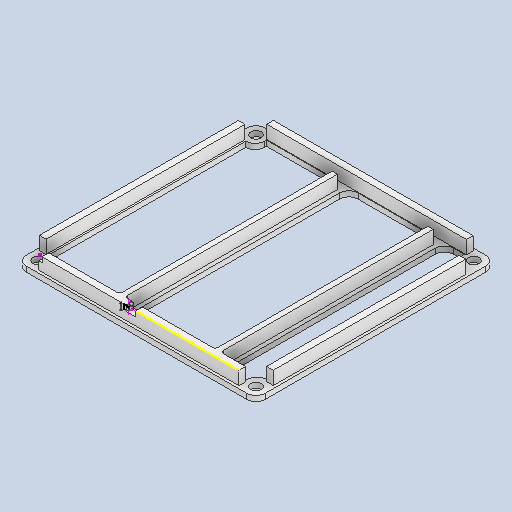
# Autodesk Inventor part: LeftCover
Saved by Autodesk Inventor 2024 (Build 280153000, 153)
## iProperties
Created: 2023-11-21
Part Number: LeftCover
Material: ABS Plastic
Document SubType Name: Modeling
Designer: G2O
Density: 1.06 g/cm^3
Appearance: Smooth - White
Author: G2O
Autodesk Inventor part; units mm, degrees
ref_plane "YZ Plane" through (0, 0, 0) normal (1, 0, 0) x (0, 1, 0)
ref_plane "XZ Plane" through (0, 0, 0) normal (0, 1, 0) x (-1, 0, 0)
ref_plane "XY Plane" through (0, 0, 0) normal (0, 0, 1) x (1, 0, 0)
sketch "Sketch1" plane through (0, 0, 0) normal (0, 1, 0) x (-1, 0, 0)
  line L0 (45, -45) -> (-45, -45)
  line L1 (-45, -45) -> (-45, 45)
  line L2 (-45, 45) -> (45, 45)
  line L3 (45, 45) -> (45, -45)
  line L4 (45, -45) -> (-45, 45) construction
  line L5 (-45, -45) -> (45, 45) construction
  point P0 (0, 0)
  dimension "d2" = 90
  dimension "d3" = 90
  constraints: 12 end point, 2 midpoint, 2 parallel, 1 horizontal, 1 perpendicular
  measures "d2" distance of L1.end L2.end
  measures "d3" distance of L0.end L1.end
extrude "Extrusion1" add sketch "Sketch1" along normal blind 2
sketch "Sketch2" plane through (0, 2, 0) normal (0, 1, 0) x (1, 0, 0)
  line L0 (45, -45) -> (45, 45) projected
  line L1 (45, 45) -> (41, 45)
  line L2 (45, 45) -> (-45, 45) projected
  circle A0 centre (41, 41) radius 2
  point P0 (0, 0)
  constraints: 2 end point, 1 centre point, 1 point on line
hole "Hole1" at (41, 2, -41) direction (0, -1, 0) diameter 4 end through all
sketch "Sketch3" plane through (0, 2, 0) normal (0, 1, 0) x (1, 0, 0)
  circle A0 centre (-41, 41) radius 2
  line L0 (-45, 45) -> (-45, -45) projected
  circle A1 centre (-41, -41) radius 2
  line L1 (45, -45) -> (45, 45) projected
  circle A2 centre (41, -41) radius 2
  point P0 (0, 0)
  dimension "d17" = 4
  dimension "d21" = 4
  constraints: 3 centre point
  measures "d17" diameter of A0
  measures "d21" diameter of A2
extrude "Extrusion2" cut sketch "Sketch3" against normal blind 2
fillet "Fillet1" radius 3.5 4 edges at (-45, 1, -45) (45, 1, -45) (45, 1, 45) (-45, 1, 45)
sketch "Sketch5" plane through (0, 2, 0) normal (0, 1, 0) x (1, 0, 0)
  line L0 (40, 40) -> (-40, 40)
  line L1 (-40, 40) -> (-40, -40)
  line L2 (-40, -40) -> (40, -40)
  line L3 (40, -40) -> (40, 40)
  line L4 (40, 40) -> (-40, -40) construction
  line L5 (-40, 40) -> (40, -40) construction
  line L6 (-9.8412, 41.25) -> (-37.3412, 41.25)
  line L7 (-37.3412, 41.25) -> (-37.3412, -41.25)
  line L8 (-37.3412, -41.25) -> (-9.8412, -41.25)
  line L9 (-9.8412, -41.25) -> (-9.8412, 41.25)
  line L10 (-9.8412, 41.25) -> (-37.3412, -41.25) construction
  line L11 (-37.3412, 41.25) -> (-9.8412, -41.25) construction
  line L12 (26.1588, 41.25) -> (-6.3412, 41.25)
  line L13 (-6.3412, 41.25) -> (-6.3412, -41.25)
  line L14 (-6.3412, -41.25) -> (26.1588, -41.25)
  line L15 (26.1588, -41.25) -> (26.1588, 41.25)
  line L16 (26.1588, 41.25) -> (-6.3412, -41.25) construction
  line L17 (-6.3412, 41.25) -> (26.1588, -41.25) construction
  line L18 (37.1268, 41.25) -> (29.6588, 41.25)
  line L19 (29.6588, 41.25) -> (29.6588, -41.25)
  line L20 (29.6588, -41.25) -> (37.1268, -41.25)
  line L21 (37.1268, -41.25) -> (37.1268, 41.25)
  line L22 (37.1268, 41.25) -> (29.6588, -41.25) construction
  line L23 (29.6588, 41.25) -> (37.1268, -41.25) construction
  line L24 (-41.5049, 41.25) -> (-37.5049, 41.25)
  line L25 (41.2164, 37.1336) -> (36.7164, 37.1336)
  line L26 (36.7164, 37.1336) -> (36.7164, -36.7164)
  line L27 (36.7164, -36.7164) -> (41.2164, -36.7164)
  line L28 (41.2164, -36.7164) -> (41.2164, 37.1336)
  line L29 (41.2164, 37.1336) -> (36.7164, -36.7164) construction
  line L30 (36.7164, 37.1336) -> (41.2164, -36.7164) construction
  line L31 (37.1268, 41.25) -> (41.1268, 41.25)
  line L32 (41.1268, 41.25) -> (41.1268, 37.25)
  point P0 (0, 0)
  point P1 (-23.5912, 0)
  point P2 (9.9088, 0)
  point P3 (33.3928, 0)
  point P4 (38.9664, 0.2086)
  point P5 (37.1268, 37.1336)
  point P6 (37.1268, 40)
  point P7 (29.6588, 40)
  point P8 (29.6588, -40)
  point P9 (37.1268, -40)
  point P10 (37.1268, -36.7164)
  dimension "d25" = 80
  dimension "d26" = 80
  dimension "d27" = 27.5
  dimension "d28" = 82.5
  dimension "d29" = 32.5
  dimension "d30" = 82.5
  dimension "d31" = 7.468
  dimension "d32" = 82.5
  dimension "d33" = 4
  dimension "d34" = 3.5
  dimension "d35" = 3.5
  dimension "d36" = 4.5
  dimension "d37" = 4
  dimension "d38" = 4
  dimension "d39" = 73.85
  constraints: 66 end point, 10 midpoint, 10 parallel, 6 horizontal, 5 perpendicular, 3 point on line, 1 vertical
  measures "d25" distance of L2.end L1.end
  measures "d26" distance of L1.end L0.end
  measures "d27" distance of L8.end L7.end
  measures "d28" distance of L6.end L7.end
  measures "d29" distance of L17.end L16.end
  measures "d30" distance of L17.start L16.end
  measures "d31" distance of L20.end L19.end
  measures "d32" distance of L18.end L19.end
  measures "d33" distance of L24.start L24.end
  measures "d34" distance between parallel lines of L13 L9
  measures "d35" distance between parallel lines of L15 L19
  measures "d36" distance of L26.end L27.end
  measures "d37" distance of L18.start L31.end
  measures "d38" distance of L31.end L32.end
  measures "d39" distance of L27.end L25.start
extrude "Extrusion4" cut sketch "Sketch5" against normal through all contours L21 L25 L26 L27 L2 L19 L0 | L0 L19 L18 L21 | L25 L28 L27 L3 | L3 L27 L21 L25 | L21 L27 L26 L25 | L15 L2 L13 L0 | L0 L13 L12 L15 | L2 L21 L20 L19 | L15 L14 L13 L2 | L9 L2 L7 L0 | L0 L7 L6 L9 | L9 L8 L7 L2
sketch "Sketch8" plane through (0, 2, 0) normal (0, 1, 0) x (1, 0, 0)
  line L0 (-45, 41.5) -> (-45, -41.5) projected
  line L1 (-45, 41.5) -> (-44, 41.5)
  line L2 (41.5, 45) -> (-41.5, 45) projected
  line L3 (-41.5, 45) -> (-41.5, 44)
  line L4 (-45, -41.5) -> (-44, -41.5)
  arc A0 (-45, -41.5) -> (-41.5, -45) centre (-41.5, -41.5) ccw projected
  line L5 (-41.5, -45) -> (-41.5, -44)
  line L6 (41.5, -45) -> (41.5, -44)
  arc A1 (41.5, -45) -> (45, -41.5) centre (41.5, -41.5) ccw projected
  line L7 (45, -41.5) -> (44, -41.5)
  arc A2 (45, 41.5) -> (41.5, 45) centre (41.5, 41.5) ccw projected
  circle A3 centre (-41, -41) radius 2 projected
  line L8 (-41, -39) -> (-41, -38)
  line L9 (-39, -41) -> (-38, -41)
  circle A4 centre (-41, 41) radius 2 projected
  line L10 (-39, 41) -> (-38, 41)
  line L11 (-41, 39) -> (-41, 38)
  circle A5 centre (41, 41) radius 2 projected
  line L12 (37.1268, 41.25) -> (37.1268, 37.1336) projected
  circle A6 centre (41, -41) radius 2 projected
  line L13 (41, -39) -> (41, -38)
  line L14 (39, -41) -> (38, -41)
  line L15 (-44, 37.3438) -> (-41.5, 37.3438)
  line L16 (-41.5, 37.3438) -> (-41.5, -37.5309)
  line L17 (-41.5, -37.5309) -> (-44, -37.5309)
  line L18 (-44, -37.5309) -> (-44, 37.3438)
  line L19 (37.5845, -44) -> (-37.7671, -44)
  line L20 (-37.7671, -44) -> (-37.7671, -41.5)
  line L21 (-37.7671, -41.5) -> (37.5845, -41.5)
  line L22 (37.5845, -41.5) -> (37.5845, -44)
  line L23 (44, 34.9904) -> (41.5, 34.9904)
  line L24 (41.5, 34.9904) -> (41.5, -37.4955)
  line L25 (41.5, -37.4955) -> (44, -37.4955)
  line L26 (44, -37.4955) -> (44, 34.9904)
  line L27 (-37.4232, 44) -> (37.7379, 44)
  line L28 (37.7379, 44) -> (37.7379, 41.5)
  line L29 (37.7379, 41.5) -> (-37.4232, 41.5)
  line L30 (-37.4232, 41.5) -> (-37.4232, 44)
  line L31 (26.1588, -41.5) -> (28.1588, -41.5)
  line L32 (28.1588, -41.5) -> (28.1588, 41.5)
  line L33 (28.1588, 41.5) -> (26.1588, 41.5)
  line L34 (26.1588, 41.5) -> (26.1588, -41.5)
  line L35 (-9.8412, -41.5) -> (-7.8412, -41.5)
  line L36 (-7.8412, -41.5) -> (-7.8412, 41.5)
  line L37 (-7.8412, 41.5) -> (-9.8412, 41.5)
  line L38 (-9.8412, 41.5) -> (-9.8412, -41.5)
  point P0 (0, 0)
  dimension "d46" = 1
  dimension "d47" = 1
  dimension "d48" = 1
  dimension "d49" = 1
  dimension "d50" = 1
  dimension "d51" = 1
  dimension "d54" = 1
  dimension "d55" = 1
  dimension "d56" = 1
  dimension "d57" = 1
  dimension "d60" = 1
  dimension "d61" = 1
  dimension "d63" = 2.5
  dimension "d64" = 2.5
  dimension "d65" = 2.5
  dimension "d72" = 2
  dimension "d73" = 2
  constraints: 72 end point, 12 horizontal, 12 parallel, 6 perpendicular, 6 point on circle, 6 vertical, 4 point on line
  measures "d46" distance of L0.start L1.end
  measures "d47" distance of L2.end L3.end
  measures "d48" distance of L0.end L4.end
  measures "d49" distance of L5.start L5.end
  measures "d50" distance of L6.start L6.end
  measures "d51" distance of L7.start L7.end
  measures "d54" distance of L8.start L8.end
  measures "d55" distance of L9.start L9.end
  measures "d56" distance of L10.start L10.end
  measures "d57" distance of L11.start L11.end
  measures "d60" distance of L13.start L13.end
  measures "d61" distance of L14.start L14.end
  measures "d63" distance of L16.end L17.end
  measures "d64" distance of L19.end L20.end
  measures "d65" distance of L25.end L24.end
  measures "d72" distance of L33.end L32.end
  measures "d73" distance of L37.end L36.end
extrude "Extrusion5" add sketch "Sketch8" along normal blind 5 contours L15 L16 L17 L18 | L19 L20 L21 L22 | L21 L34 L29 L32 | L38 L29 L36 L21 | L29 L30 L27 L28 | L26 L25 L24 L23
fillet "Fillet3" radius 3.5 1 edges at (37.1268, 1, 36.7164)
fillet "Fillet4" radius 3.5 8 edges at (-6.3412, 1, 41.25) (-6.3412, 1, -41.25) (29.6588, 1, -41.25) (29.6588, 1, 41.25) (26.1588, 1, -41.25) (-9.8412, 1, -41.25) (26.1588, 1, 41.25) (-9.8412, 1, 41.25)
fillet "Fillet7" radius 1 4 edges at (-7.8412, 4.5, 41.5) (28.1588, 4.5, 41.5) (26.1588, 4.5, 41.5) (-9.8412, 4.5, 41.5)
sketch "Sketch10" plane through (0, 0, 0) normal (0, -1, 0) x (1, 0, 0)
  line L0 (-37.3412, -41.25) -> (-37.3412, 41.25) projected
  line L1 (-37.3412, 37.75) -> (-40.8412, 37.75)
  line L2 (-40.8412, 37.75) -> (-40.8412, -37)
  line L3 (-40.8412, -37) -> (-37.3412, -37)
  line L4 (-37.3412, -37) -> (-37.3412, 37.75)
  point P0 (0, 0)
  point P1 (-37.3412, -37.75)
  dimension "d78" = 3.5
  constraints: 8 end point, 2 parallel, 1 horizontal, 1 perpendicular
  measures "d78" distance of L3.end L2.end
extrude "Extrusion6" cut sketch "Sketch10" against normal through all
fillet "Fillet8" radius 3.5 1 edges at (-37.3412, 1, -37)
fillet "Fillet11" radius 3.5 2 edges at (37.1268, 1, -37.1336) (-37.3412, 1, 37.75)
sketch "Sketch19" plane through (-37.7671, 2, 44) normal (0, 0, 1) x (1, 0, 0)
  line L0 (75.3516, 0) -> (0, 0) projected
  line L1 (0, 5) -> (75.3516, 5) projected
  line L2 (0, 0) -> (0, 5) projected
  line L3 (0, 5) -> (0, 3)
  line L4 (0, 3) -> (1.2108, 3)
  line L5 (1.2108, 3) -> (1.2108, 5)
  line L6 (1.2108, 5) -> (0, 5)
  line L7 (0, 5) -> (0, 3)
  point P0 (37.7671, -2)
  dimension "d90" = 2
  dimension "d106" = 1.2108
  constraints: 10 end point, 2 parallel, 2 point on line, 1 horizontal, 1 perpendicular
  measures "d90" distance of L1.start L3.end
  measures "d106" distance of L3.end L4.end
extrude "Extrusion7" cut sketch "Sketch19" against normal blind 3
sketch "Sketch21" plane through (25.1588, 2, 41.5) normal (0, 0, -1) x (-1, 0, 0)
  line L0 (32, 0) -> (0, 0) projected
  line L1 (0, 5) -> (32, 5) projected
  line L2 (28.159, 5) -> (29.959, 5)
  line L3 (29.959, 5) -> (29.959, 4)
  line L4 (28.159, 5) -> (26.359, 5)
  line L5 (29.959, 5) -> (26.359, 5)
  line L6 (26.359, 5) -> (26.359, 3)
  line L7 (26.359, 3) -> (29.959, 3)
  line L8 (29.959, 3) -> (29.959, 5)
  point P0 (25.1588, -2)
  point P1 (29.959, 4)
  dimension "d102" = 1.8
  dimension "d103" = 1
  dimension "d104" = 1.8
  dimension "d105" = 2
  constraints: 14 end point, 3 point on line, 2 parallel, 1 horizontal, 1 perpendicular, 1 vertical
  measures "d102" distance of L2.start L2.end
  measures "d103" distance of L2.end L3.end
  measures "d104" distance of L2.start L4.end
  measures "d105" distance of L6.end L5.end
extrude "Extrusion8" cut sketch "Sketch21" against normal up to surface (2.5 mm away)
sketch "Sketch22" plane through (-9.8412, 2, -41.5) normal (-1, 0, 0) x (0, 0, 1)
  line L0 (0, 5) -> (82, 5) projected
  line L1 (0, 5) -> (3, 5)
  line L2 (3.75, 0) -> (0, 0) projected
  line L3 (3, 5) -> (0, 5)
  line L4 (0, 5) -> (0, 0)
  line L5 (0, 0) -> (3, 0)
  line L6 (3, 0) -> (3, 5)
  point P0 (41.5, -2)
  point P1 (3, 0)
  dimension "d98" = 3
  constraints: 10 end point, 2 parallel, 1 horizontal, 1 perpendicular, 1 point on line
  measures "d98" distance of L0.start L1.end
extrude "Extrusion9" cut sketch "Sketch22" against normal up to surface (38 mm away)
sketch "Sketch23" plane through (-37.7671, 2, 44) normal (0, 0, 1) x (1, 0, 0)
  line L0 (33.7518, 5) -> (31.9518, 5)
  line L1 (36.5669, 5) -> (75.3516, 5) projected
  line L2 (31.9518, 5) -> (31.9518, 3.1171)
  point P0 (37.7671, -2)
  point P1 (0.3379, 5)
  dimension "d101" = 1.8
  constraints: 4 end point, 1 point on line, 1 vertical
  measures "d101" distance of L0.start L0.end
sketch "Sketch24" plane through (-37.7671, 2, 44) normal (0, 0, 1) x (1, 0, 0)
  point P0 (37.7671, -2)
body "Solid1"
